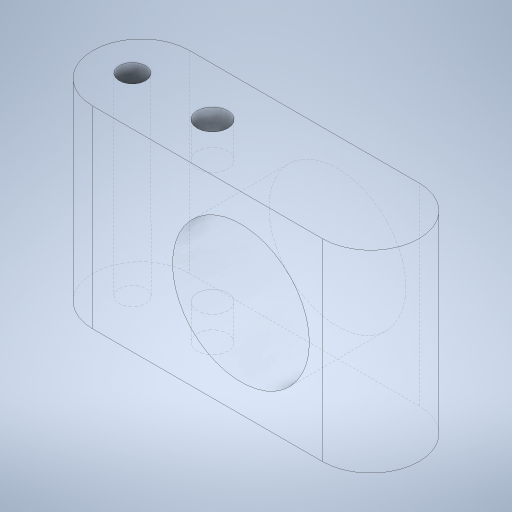
# Autodesk Inventor part: Reworked - PlateArmClip22mm
Saved by Autodesk Inventor 2023 (Build 270158000, 158)
## iProperties
Created: 2022-12-05
Part Number: Reworked - PlateArmClip22mm
Material: Generic
Document SubType Name: Modeling
Designer: Administrator
Density: 1 g/cm^3
Appearance: Default
Author: Administrator
Autodesk Inventor part; units mm, degrees
ref_plane "YZ Plane" through (0, 0, 0) normal (1, 0, 0) x (0, 1, 0)
ref_plane "XZ Plane" through (0, 0, 0) normal (0, 1, 0) x (-1, 0, 0)
ref_plane "XY Plane" through (0, 0, 0) normal (0, 0, 1) x (1, 0, 0)
sketch "Sketch1" plane through (0, 0, 0) normal (0, 0, 1) x (1, 0, 0)
  circle A0 centre (0, 0) radius 7.8
  line L0 (0, 0) -> (-8.735, 0) construction
  line L1 (0, 0) -> (-17.865, 0) construction
  line L2 (-8.735, 0) -> (-8.735, 11) construction
  line L3 (-8.735, 0) -> (-8.735, -11) construction
  line L4 (-17.865, 0) -> (-17.865, -11) construction
  line L5 (-17.865, 0) -> (-17.865, 11) construction
  line L6 (7.8, 0) -> (14.8, 0) construction
  line L7 (-17.865, 0) -> (-22.365, 0) construction
  line L8 (-22.365, -11) -> (14.8, -11)
  line L9 (14.8, -11) -> (14.8, 11)
  line L10 (14.8, 11) -> (-22.365, 11)
  line L11 (-22.365, 11) -> (-22.365, -11)
  dimension "d0" = 15.6
  dimension "d1" = 8.735
  dimension "d2" = 17.865
  dimension "d3" = 11
  dimension "d4" = 11
  dimension "d5" = 11
  dimension "d6" = 11
  dimension "d7" = 7
  dimension "d8" = 4.5
  dimension "d23" = 37.165
  constraints: 24 end point, 5 horizontal, 4 vertical, 2 parallel, 1 coincident, 1 horizontal alignment, 1 perpendicular, 2 other
  measures "d1" distance of L0.start L0.end
  measures "d2" distance of L0.start L1.end
  measures "d3" distance of L0.end L2.end
  measures "d4" distance of L0.end L3.end
  measures "d5" distance of L1.end L4.end
  measures "d6" distance of L1.end L5.end
  measures "d7" distance of L6.start L6.end
  measures "d8" distance of L1.end L7.end
  measures "d23" distance of L9.end L10.end
extrude "Extrusion1" add sketch "Sketch1" along normal mid plane 11
sketch "Sketch2" plane through (-22.365, 11, 5.5) normal (0, 1, 0) x (1, 0, 0)
  line L0 (0, 11) -> (0, 0) projected
  line L1 (0, 5.5) -> (4.5, 5.5)
  line L2 (4.5, 5.5) -> (13.63, 5.5)
  circle A0 centre (4.5, 5.5) radius 1.5
  circle A1 centre (13.63, 5.5) radius 1.75
  point P0 (22.365, 5.5)
  dimension "d11" = 4.5
  dimension "d13" = 9.13
  dimension "d14" = 3
  dimension "d15" = 3.5
  constraints: 4 end point, 2 centre point, 2 coincident, 2 horizontal, 1 midpoint
  measures "d11" distance of L1.start L1.end
  measures "d13" distance of L1.end L2.end
  measures "d14" diameter of A0
  measures "d15" diameter of A1
extrude "Extrusion2" cut sketch "Sketch2" against normal up to next contours A0 L2 L1 | L1 L2 A0
extrude "Extrusion3" cut sketch "Sketch2" against normal blind 4 contours A1
sketch "Sketch3" plane through (-22.365, -11, 5.5) normal (0, -1, 0) x (1, 0, 0)
  circle A0 centre (13.63, -5.5) radius 1.75 projected
  circle A1 centre (13.63, -5.5) radius 1.75
  point P0 (22.365, -5.5)
  constraints: 1 centre point, 1 coincident
extrude "Extrusion4" cut sketch "Sketch3" against normal blind 4
fillet "Fillet1" radius 5.5 4 edges at (-22.365, 0, 5.5) (14.8, 0, 5.5) (14.8, 0, -5.5) (-22.365, 0, -5.5)
equation "\"d23\" = d2 + d7 + 0.5 * d0 + d8"
body "Solid1"
